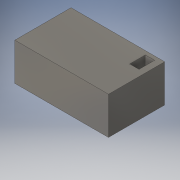
# Autodesk Inventor part: Box
Saved by Autodesk Inventor 2016 (Build 200138000, 138)
## iProperties
Created: 2015-11-30
Part Number: Box
Material: Generic
Document SubType Name: Modeling
Designer: Javier
Density: 1 g/cm^3
Appearance: Diamond Plate
Author: Javier
Autodesk Inventor part; units mm, degrees
ref_plane "YZ Plane" through (0, 0, 0) normal (1, 0, 0) x (0, 1, 0)
sketch "Sketch1" plane through (0, 0, 0) normal (0, 1, 0) x (-1, 0, 0)
  line L0 (381, -209.55) -> (-381, -209.55)
  line L1 (-381, -209.55) -> (-381, 247.65)
  line L2 (-381, 247.65) -> (381, 247.65)
  line L3 (381, 247.65) -> (381, -209.55)
  point P0 (0, 0)
  dimension "d0" = 762
  constraints: 8 end point, 2 parallel, 1 horizontal, 1 perpendicular
  measures "d0" distance between parallel lines of L1 L3
extrude "Extrusion1" add sketch "Sketch1" along normal blind 304.8
ref_plane "Work Plane1" through (0, 304.8, 0) normal (0, 1, 0) x (-1, 0, 0)
sketch "Sketch2" plane through (0, 304.8, 0) normal (0, 1, 0) x (-1, 0, 0)
  line L0 (-254, -51.5336) -> (-330.2, -51.5336)
  line L1 (-330.2, -51.5336) -> (-330.2, -178.5336)
  line L2 (-330.2, -178.5336) -> (-254, -178.5336)
  line L3 (-254, -178.5336) -> (-254, -51.5336)
  line L4 (-381, 247.65) -> (-381, -209.55) projected
  line L5 (381, 247.65) -> (-381, 247.65) projected
  point P0 (0, 0)
  dimension "d6" = 127
  dimension "d7" = 76.2
  constraints: 8 end point, 2 parallel, 1 horizontal, 1 perpendicular
  measures "d6" distance of L0.start L2.end
  measures "d7" distance between parallel lines of L1 L3
extrude "Extrusion2" cut sketch "Sketch2" against normal blind 304.8
ref_plane "Work Plane2" through (0, 0, -213.36) normal (0, 0, 1) x (1, 0, 0)
sketch "Sketch3" plane through (0, 0, -213.36) normal (0, 0, 1) x (1, 0, 0)
  point P0 (0, 0)
sketch "Sketch4" plane through (0, 0, -213.36) normal (0, 0, 1) x (1, 0, 0)
  line L0 (-123.0782, 274.0785) -> (124.5718, 274.0785) construction
  line L1 (124.5718, 274.0785) -> (124.5718, 26.4285) construction
  line L2 (124.5718, 26.4285) -> (-123.0782, 26.4285) construction
  line L3 (-123.0782, 26.4285) -> (-123.0782, 274.0785) construction
  point P0 (0, 0)
  constraints: 2 other
body "Solid1"
